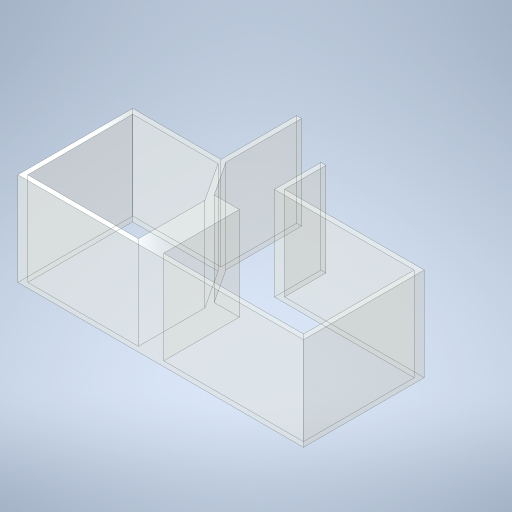
# Autodesk Inventor part: Existing_Kitchen_And_Dining_Room
Saved by Autodesk Inventor 2024 (Build 280153000, 153)
## iProperties
Created: 2023-04-15
Part Number: Existing_Kitchen_And_Dining_Room
Material: Glass
Document SubType Name: Modeling
Designer: Tom
Density: 2.18 g/cm^3
Appearance: Clear
Author: Tom
Autodesk Inventor part; units mm, degrees
ref_plane "YZ Plane" through (0, 0, 0) normal (1, 0, 0) x (0, 1, 0)
ref_plane "XZ Plane" through (0, 0, 0) normal (0, 1, 0) x (-1, 0, 0)
ref_plane "XY Plane" through (0, 0, 0) normal (0, 0, 1) x (1, 0, 0)
sketch "Sketch1" plane through (0, 0, 0) normal (0, 1, 0) x (-1, 0, 0)
  line L0 (0, 0) -> (0, -2743.2)
  line L1 (0, -2743.2) -> (-2235.2, -2743.2)
  line L2 (0, 0) -> (-7213.6, 0)
  line L3 (-2895.6, 0) -> (-3556, 0)
  line L4 (-3556, 0) -> (-3556, -1981.2)
  line L5 (-3556, -1981.2) -> (-2895.6, -1981.2)
  line L6 (-2895.6, -1738.4107) -> (-2895.6, 0)
  line L7 (-7213.6, 0) -> (-7213.6, -2895.6)
  line L8 (-7213.6, -2895.6) -> (-3556, -2895.6)
  line L9 (-2176.9542, -2876.55) -> (130.175, -2876.55)
  line L10 (130.175, -2876.55) -> (130.175, 130.175)
  line L11 (130.175, 130.175) -> (-7343.775, 130.175)
  line L12 (-7343.775, 130.175) -> (-7343.775, -3028.95)
  line L13 (-7343.775, -3028.95) -> (-3686.175, -3028.95)
  line L14 (-3556, -4114.8) -> (-3556, -2895.6)
  line L15 (-2307.1292, -2876.55) -> (-2895.6, -1981.2)
  line L16 (-2235.2, -2743.2) -> (-2895.6, -1738.4107)
  line L17 (-2176.9542, -2876.55) -> (-2176.9542, -4857.75)
  line L18 (-2176.9542, -4857.75) -> (-2307.1292, -4857.75)
  line L19 (-2307.1292, -4857.75) -> (-2307.1292, -2876.55)
  line L20 (-3686.175, -3028.95) -> (-3686.175, -4114.8)
  line L21 (-3686.175, -4114.8) -> (-3556, -4114.8)
  point P0 (-2601.3646, -2428.875)
  dimension "d1" = 2743.2
  dimension "d3" = 7213.6
  dimension "d4" = 2895.6
  dimension "d5" = 660.4
  dimension "d6" = 1981.2
  dimension "d7" = 914.4
  dimension "d8" = 3657.6
  dimension "d10" = 130.175
  dimension "d11" = 130.175
  dimension "d12" = 130.175
  dimension "d13" = 133.35
  dimension "d16" = 133.35
  dimension "d21" = 1219.2
  dimension "d22" = 130.175
  dimension "d24" = 2235.2
  dimension "d25" = 1981.2
  dimension "d26" = 133.35
  dimension "d27" = 130.175
  dimension "d28" = 58.2458
  constraints: 44 end point, 10 perpendicular, 4 parallel, 3 horizontal, 2 point on line, 2 vertical, 1 midpoint
  measures "d1" distance of L0.start L0.end
  measures "d3" distance of L0.start L2.end
  measures "d4" distance between parallel lines of L6 L0
  measures "d5" distance between parallel lines of L4 L6
  measures "d6" distance of L5.end L3.start
  measures "d7" distance between parallel lines of L8 L5
  measures "d8" distance of L7.end L8.end
  measures "d10" distance between parallel lines of L10 L0
  measures "d11" distance between parallel lines of L11 L2
  measures "d12" distance between parallel lines of L7 L12
  measures "d13" distance between parallel lines of L8 L13
  measures "d16" distance between parallel lines of L9 L1
  measures "d21" distance of L14.start L8.end
  measures "d22" distance between parallel lines of L20 L14
  measures "d24" distance of L0.end L1.end
  measures "d25" distance of L18.end L15.start
  measures "d26" distance between parallel lines of L15 L16
  measures "d27" distance between parallel lines of L17 L19
  measures "d28" distance from line of L17 L1.end
extrude "Extrusion1" add sketch "Sketch1" along normal blind 2438.4
body "Solid1"
